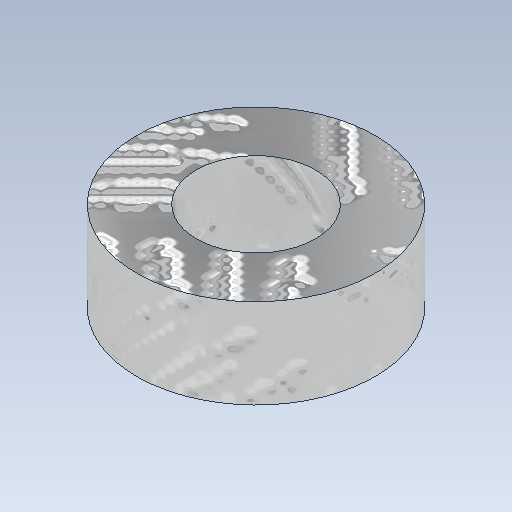
# Autodesk Inventor part: ハンド_ベアリング_4-8
Saved by Autodesk Inventor 2020.3 (Build 243373000, 373)
## iProperties
Created: 2020-06-01
Part Number: ハンド_ベアリング_4-8
Material: 鋼、炭素鋼
Document SubType Name: Modeling
Designer: totot
Density: 7.85 g/cm^3
Appearance: プレート - 青
Mass: 0.887814 g
Surface Area: 1.88496 cm^2
Volume: 0.113097 cm^3
Author: totot
Autodesk Inventor part; units mm, degrees
ref_plane "YZ Plane" through (0, 0, 0) normal (1, 0, 0) x (0, 1, 0)
ref_plane "XZ Plane" through (0, 0, 0) normal (0, 1, 0) x (-1, 0, 0)
ref_plane "XY Plane" through (0, 0, 0) normal (0, 0, 1) x (1, 0, 0)
sketch "スケッチ1" plane through (0, 0, 0) normal (0, 1, 0) x (-1, 0, 0)
  circle A0 centre (0, 0) radius 4
  circle A1 centre (0, 0) radius 2
  dimension "d0" = 8
  dimension "d1" = 4
  constraints: 2 centre point, 2 coincident
  measures "d0" diameter of A0
  measures "d1" diameter of A1
extrude "押し出し1" add sketch "スケッチ1" along normal blind 3
